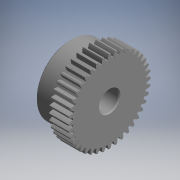
# Autodesk Inventor part: PS1-40_On
Saved by Autodesk Inventor 2017.3 (Build 213256000, 256)
## iProperties
Part Number: PS1-40_On
Material: Generic
Catalog Web Link: www.cadenas.de
Description: Plastic Spur Gears (PS)-
Vendor: KHK
Document SubType Name: Modeling
Designer: partserver
Manufacturer: KHK
Mass: 20.4717 g
Surface Area: 64.8877 cm^2
Volume: 20.4717 cm^3
Density: 1 g/cm^3
Appearance: PSOLRGB-175-175-175
Category: PARTsolutions
Company: KHK
Title: PS1-40
Author: Cadenas PARTsolutions
PSOL_IDENT_0: {$CADENAS_DATA\23d-libs\khk\spur_gears\plastic_spur_gears_ps.prj},178 {VTYP=3D},{NB=PS1-40_On},{LINA=
PSOL_IDENT_1: PS1-40},{NN=Plastic Spur Gears (PS)},{DATE=10.04.2020 06:07:24},{GEOMDATE=05.07.2019 08:26:52},{VERS
PSOL_IDENT_2: ION=},{LINEID=150},{WBVAR=TOOTH},{WBNUMERIC=}  {NB=PS1-40_On},{LINA=PS1-40},{KT=DUMMY},{CN=PS1-40},{
PSOL_IDENT_3: M=1},{MX=1.000},{Z=40},{S=S1},{A=10},{B=35},{C=40.0},{D=42.0},{E=10},{F=10},{G=20},{K=0},{KD=0.0},{M
PSOL_IDENT_4: 1=0},{SCSX=0},{J=0.0},{WMF=S1003.WMF},{R=1.0},{N=0.5},{L=0.1},{L2=0.5},{CBD1=0.0},{CBD2=0.0},{TOOTH=
PSOL_IDENT_5: On}
NB: PS1-40_On
NN: Plastic Spur Gears (PS)
NBSYN: $CN._$TOOTH.
LINA: PS1-40
CATALOG: KHK
CN: PS1-40
M: 1
Z: 40
S: S1
A: 10
B: 35
C: 40
D: 42
E: 10
F: 10
G: 20
K: 0
KD: 0
M1: 0
J: 0
TOOTH: On
SUPPLIER: KHK
ARTICLENO: PS1-40_On
BOMINFO: PS1-40
CREATOR: CADENAS GmbH
Autodesk Inventor part; units mm, degrees
ref_plane "YZ Plane" through (0, 0, 0) normal (1, 0, 0) x (0, 1, 0)
ref_plane "XZ Plane" through (0, 0, 0) normal (0, 1, 0) x (-1, 0, 0)
ref_plane "XY Plane" through (0, 0, 0) normal (0, 0, 1) x (1, 0, 0)
sketch "Sketch_8" plane through (0, 0, 0) normal (0, 0, 1) x (1, 0, 0)
  line L0 (20, 0) -> (0, 0)
  line L1 (0, 5.5) -> (0.5, 5)
  line L2 (0.5, 5) -> (19.5, 5)
  line L3 (19.5, 5) -> (20, 5.5)
  line L4 (20, 5.5) -> (20, 17)
  line L5 (20, 17) -> (19.5, 17.5)
  line L6 (19.5, 17.5) -> (11, 17.5)
  arc A0 (10, 18.5) -> (11, 17.5) centre (11, 18.5) ccw
  line L7 (10, 18.5) -> (10, 20.9)
  line L8 (10, 20.9) -> (9.9, 21)
  line L9 (9.9, 21) -> (0.1, 21)
  line L10 (0.1, 21) -> (0, 20.9)
  line L11 (0, 20.9) -> (0, 5.5)
  constraints: 24 end point, 2 point on circle, 1 centre point
revolve "Revolution1" add sketch "Sketch_8" angle 360 about axis through (20, 0, 0) along (1, 0, 0)
sketch "Sketch_11" plane through (0, 0, 0) normal (1, 0, 0) x (0, 1, 0)
  line L0 (42, 42) -> (-42, 42)
  line L1 (-42, 42) -> (-42, -42)
  line L2 (-42, -42) -> (42, -42)
  line L3 (42, -42) -> (42, 42)
  arc A0 (0.3299, 20.9974) -> (-0.3299, 20.9974) centre (0, 0) ccw
  arc A1 (-0.3299, 20.9974) -> (-1.0303, 18.7217) centre (4.9404, 18.1296) ccw
  arc A2 (-1.0303, 18.7217) -> (-1.9111, 18.6524) centre (0, 0) ccw
  arc A3 (-1.9111, 18.6524) -> (-2.9589, 20.7905) centre (-7.7157, 17.1335) ccw
  arc A4 (-2.9589, 20.7905) -> (-3.6105, 20.6873) centre (0, 0) ccw
  arc A5 (-3.6105, 20.6873) -> (-3.9463, 18.33) centre (2.0435, 18.6792) ccw
  arc A6 (-3.9463, 18.33) -> (-4.8054, 18.1238) centre (0, 0) ccw
  arc A7 (-4.8054, 18.1238) -> (-6.1748, 20.0717) centre (-10.3009, 15.7156) ccw
  arc A8 (-6.1748, 20.0717) -> (-6.8023, 19.8678) centre (0, 0) ccw
  arc A9 (-6.8023, 19.8678) -> (-6.7652, 17.487) centre (-0.9038, 18.7689) ccw
  arc A10 (-6.7652, 17.487) -> (-7.5814, 17.1489) centre (0, 0) ccw
  arc A11 (-7.5814, 17.1489) -> (-9.2387, 18.8586) centre (-12.6326, 13.9107) ccw
  arc A12 (-9.2387, 18.8586) -> (-9.8265, 18.5591) centre (0, 0) ccw
  arc A13 (-9.8265, 18.5591) -> (-9.4175, 16.2134) centre (-3.8287, 18.3965) ccw
  arc A14 (-9.4175, 16.2134) -> (-10.1708, 15.7518) centre (0, 0) ccw
  arc A15 (-10.1708, 15.7518) -> (-12.0751, 17.1811) centre (-14.6532, 11.7632) ccw
  arc A16 (-12.0751, 17.1811) -> (-12.6088, 16.7934) centre (0, 0) ccw
  arc A17 (-12.6088, 16.7934) -> (-11.8379, 14.5405) centre (-6.6594, 17.571) ccw
  arc A18 (-11.8379, 14.5405) -> (-12.5097, 13.9668) centre (0, 0) ccw
  arc A19 (-12.5097, 13.9668) -> (-14.6142, 15.0807) centre (-16.3129, 9.3262) ccw
  arc A20 (-14.6142, 15.0807) -> (-15.0807, 14.6142) centre (0, 0) ccw
  arc A21 (-15.0807, 14.6142) -> (-13.9668, 12.5097) centre (-9.3262, 16.3129) ccw
  arc A22 (-13.9668, 12.5097) -> (-14.5405, 11.8379) centre (0, 0) ccw
  arc A23 (-14.5405, 11.8379) -> (-16.7934, 12.6088) centre (-17.571, 6.6594) ccw
  arc A24 (-16.7934, 12.6088) -> (-17.1811, 12.0751) centre (0, 0) ccw
  arc A25 (-17.1811, 12.0751) -> (-15.7518, 10.1708) centre (-11.7632, 14.6532) ccw
  arc A26 (-15.7518, 10.1708) -> (-16.2134, 9.4175) centre (0, 0) ccw
  arc A27 (-16.2134, 9.4175) -> (-18.5591, 9.8265) centre (-18.3965, 3.8287) ccw
  arc A28 (-18.5591, 9.8265) -> (-18.8586, 9.2387) centre (0, 0) ccw
  arc A29 (-18.8586, 9.2387) -> (-17.1489, 7.5814) centre (-13.9107, 12.6326) ccw
  arc A30 (-17.1489, 7.5814) -> (-17.487, 6.7652) centre (0, 0) ccw
  arc A31 (-17.487, 6.7652) -> (-19.8678, 6.8023) centre (-18.7689, 0.9038) ccw
  arc A32 (-19.8678, 6.8023) -> (-20.0717, 6.1748) centre (0, 0) ccw
  arc A33 (-20.0717, 6.1748) -> (-18.1238, 4.8054) centre (-15.7156, 10.3009) ccw
  arc A34 (-18.1238, 4.8054) -> (-18.33, 3.9463) centre (0, 0) ccw
  arc A35 (-18.33, 3.9463) -> (-20.6873, 3.6105) centre (-18.6792, -2.0435) ccw
  arc A36 (-20.6873, 3.6105) -> (-20.7905, 2.9589) centre (0, 0) ccw
  arc A37 (-20.7905, 2.9589) -> (-18.6524, 1.9111) centre (-17.1335, 7.7157) ccw
  arc A38 (-18.6524, 1.9111) -> (-18.7217, 1.0303) centre (0, 0) ccw
  arc A39 (-18.7217, 1.0303) -> (-20.9974, 0.3299) centre (-18.1296, -4.9404) ccw
  arc A40 (-20.9974, 0.3299) -> (-20.9974, -0.3299) centre (0, 0) ccw
  arc A41 (-20.9974, -0.3299) -> (-18.7217, -1.0303) centre (-18.1296, 4.9404) ccw
  arc A42 (-18.7217, -1.0303) -> (-18.6524, -1.9111) centre (0, 0) ccw
  arc A43 (-18.6524, -1.9111) -> (-20.7905, -2.9589) centre (-17.1335, -7.7157) ccw
  arc A44 (-20.7905, -2.9589) -> (-20.6873, -3.6105) centre (0, 0) ccw
  arc A45 (-20.6873, -3.6105) -> (-18.33, -3.9463) centre (-18.6792, 2.0435) ccw
  arc A46 (-18.33, -3.9463) -> (-18.1238, -4.8054) centre (0, 0) ccw
  arc A47 (-18.1238, -4.8054) -> (-20.0717, -6.1748) centre (-15.7156, -10.3009) ccw
  arc A48 (-20.0717, -6.1748) -> (-19.8678, -6.8023) centre (0, 0) ccw
  arc A49 (-19.8678, -6.8023) -> (-17.487, -6.7652) centre (-18.7689, -0.9038) ccw
  arc A50 (-17.487, -6.7652) -> (-17.1489, -7.5814) centre (0, 0) ccw
  arc A51 (-17.1489, -7.5814) -> (-18.8586, -9.2387) centre (-13.9107, -12.6326) ccw
  arc A52 (-18.8586, -9.2387) -> (-18.5591, -9.8265) centre (0, 0) ccw
  arc A53 (-18.5591, -9.8265) -> (-16.2134, -9.4175) centre (-18.3965, -3.8287) ccw
  arc A54 (-16.2134, -9.4175) -> (-15.7518, -10.1708) centre (0, 0) ccw
  arc A55 (-15.7518, -10.1708) -> (-17.1811, -12.0751) centre (-11.7632, -14.6532) ccw
  arc A56 (-17.1811, -12.0751) -> (-16.7934, -12.6088) centre (0, 0) ccw
  arc A57 (-16.7934, -12.6088) -> (-14.5405, -11.8379) centre (-17.571, -6.6594) ccw
  arc A58 (-14.5405, -11.8379) -> (-13.9668, -12.5097) centre (0, 0) ccw
  arc A59 (-13.9668, -12.5097) -> (-15.0807, -14.6142) centre (-9.3262, -16.3129) ccw
  arc A60 (-15.0807, -14.6142) -> (-14.6142, -15.0807) centre (0, 0) ccw
  arc A61 (-14.6142, -15.0807) -> (-12.5097, -13.9668) centre (-16.3129, -9.3262) ccw
  arc A62 (-12.5097, -13.9668) -> (-11.8379, -14.5405) centre (0, 0) ccw
  arc A63 (-11.8379, -14.5405) -> (-12.6088, -16.7934) centre (-6.6594, -17.571) ccw
  arc A64 (-12.6088, -16.7934) -> (-12.0751, -17.1811) centre (0, 0) ccw
  arc A65 (-12.0751, -17.1811) -> (-10.1708, -15.7518) centre (-14.6532, -11.7632) ccw
  arc A66 (-10.1708, -15.7518) -> (-9.4175, -16.2134) centre (0, 0) ccw
  arc A67 (-9.4175, -16.2134) -> (-9.8265, -18.5591) centre (-3.8287, -18.3965) ccw
  arc A68 (-9.8265, -18.5591) -> (-9.2387, -18.8586) centre (0, 0) ccw
  arc A69 (-9.2387, -18.8586) -> (-7.5814, -17.1489) centre (-12.6326, -13.9107) ccw
  arc A70 (-7.5814, -17.1489) -> (-6.7652, -17.487) centre (0, 0) ccw
  arc A71 (-6.7652, -17.487) -> (-6.8023, -19.8678) centre (-0.9038, -18.7689) ccw
  arc A72 (-6.8023, -19.8678) -> (-6.1748, -20.0717) centre (0, 0) ccw
  arc A73 (-6.1748, -20.0717) -> (-4.8054, -18.1238) centre (-10.3009, -15.7156) ccw
  arc A74 (-4.8054, -18.1238) -> (-3.9463, -18.33) centre (0, 0) ccw
  arc A75 (-3.9463, -18.33) -> (-3.6105, -20.6873) centre (2.0435, -18.6792) ccw
  arc A76 (-3.6105, -20.6873) -> (-2.9589, -20.7905) centre (0, 0) ccw
  arc A77 (-2.9589, -20.7905) -> (-1.9111, -18.6524) centre (-7.7157, -17.1335) ccw
  arc A78 (-1.9111, -18.6524) -> (-1.0303, -18.7217) centre (0, 0) ccw
  arc A79 (-1.0303, -18.7217) -> (-0.3299, -20.9974) centre (4.9404, -18.1296) ccw
  arc A80 (-0.3299, -20.9974) -> (0.3299, -20.9974) centre (0, 0) ccw
  arc A81 (0.3299, -20.9974) -> (1.0303, -18.7217) centre (-4.9404, -18.1296) ccw
  arc A82 (1.0303, -18.7217) -> (1.9111, -18.6524) centre (0, 0) ccw
  arc A83 (1.9111, -18.6524) -> (2.9589, -20.7905) centre (7.7157, -17.1335) ccw
  arc A84 (2.9589, -20.7905) -> (3.6105, -20.6873) centre (0, 0) ccw
  arc A85 (3.6105, -20.6873) -> (3.9463, -18.33) centre (-2.0435, -18.6792) ccw
  arc A86 (3.9463, -18.33) -> (4.8054, -18.1238) centre (0, 0) ccw
  arc A87 (4.8054, -18.1238) -> (6.1748, -20.0717) centre (10.3009, -15.7156) ccw
  arc A88 (6.1748, -20.0717) -> (6.8023, -19.8678) centre (0, 0) ccw
  arc A89 (6.8023, -19.8678) -> (6.7652, -17.487) centre (0.9038, -18.7689) ccw
  arc A90 (6.7652, -17.487) -> (7.5814, -17.1489) centre (0, 0) ccw
  arc A91 (7.5814, -17.1489) -> (9.2387, -18.8586) centre (12.6326, -13.9107) ccw
  arc A92 (9.2387, -18.8586) -> (9.8265, -18.5591) centre (0, 0) ccw
  arc A93 (9.8265, -18.5591) -> (9.4175, -16.2134) centre (3.8287, -18.3965) ccw
  arc A94 (9.4175, -16.2134) -> (10.1708, -15.7518) centre (0, 0) ccw
  arc A95 (10.1708, -15.7518) -> (12.0751, -17.1811) centre (14.6532, -11.7632) ccw
  arc A96 (12.0751, -17.1811) -> (12.6088, -16.7934) centre (0, 0) ccw
  arc A97 (12.6088, -16.7934) -> (11.8379, -14.5405) centre (6.6594, -17.571) ccw
  arc A98 (11.8379, -14.5405) -> (12.5097, -13.9668) centre (0, 0) ccw
  arc A99 (12.5097, -13.9668) -> (14.6142, -15.0807) centre (16.3129, -9.3262) ccw
  arc A100 (14.6142, -15.0807) -> (15.0807, -14.6142) centre (0, 0) ccw
  arc A101 (15.0807, -14.6142) -> (13.9668, -12.5097) centre (9.3262, -16.3129) ccw
  arc A102 (13.9668, -12.5097) -> (14.5405, -11.8379) centre (0, 0) ccw
  arc A103 (14.5405, -11.8379) -> (16.7934, -12.6088) centre (17.571, -6.6594) ccw
  arc A104 (16.7934, -12.6088) -> (17.1811, -12.0751) centre (0, 0) ccw
  arc A105 (17.1811, -12.0751) -> (15.7518, -10.1708) centre (11.7632, -14.6532) ccw
  arc A106 (15.7518, -10.1708) -> (16.2134, -9.4175) centre (0, 0) ccw
  arc A107 (16.2134, -9.4175) -> (18.5591, -9.8265) centre (18.3965, -3.8287) ccw
  arc A108 (18.5591, -9.8265) -> (18.8586, -9.2387) centre (0, 0) ccw
  arc A109 (18.8586, -9.2387) -> (17.1489, -7.5814) centre (13.9107, -12.6326) ccw
  arc A110 (17.1489, -7.5814) -> (17.487, -6.7652) centre (0, 0) ccw
  arc A111 (17.487, -6.7652) -> (19.8678, -6.8023) centre (18.7689, -0.9038) ccw
  arc A112 (19.8678, -6.8023) -> (20.0717, -6.1748) centre (0, 0) ccw
  arc A113 (20.0717, -6.1748) -> (18.1238, -4.8054) centre (15.7156, -10.3009) ccw
  arc A114 (18.1238, -4.8054) -> (18.33, -3.9463) centre (0, 0) ccw
  arc A115 (18.33, -3.9463) -> (20.6873, -3.6105) centre (18.6792, 2.0435) ccw
  arc A116 (20.6873, -3.6105) -> (20.7905, -2.9589) centre (0, 0) ccw
  arc A117 (20.7905, -2.9589) -> (18.6524, -1.9111) centre (17.1335, -7.7157) ccw
  arc A118 (18.6524, -1.9111) -> (18.7217, -1.0303) centre (0, 0) ccw
  arc A119 (18.7217, -1.0303) -> (20.9974, -0.3299) centre (18.1296, 4.9404) ccw
  arc A120 (20.9974, -0.3299) -> (20.9974, 0.3299) centre (0, 0) ccw
  arc A121 (20.9974, 0.3299) -> (18.7217, 1.0303) centre (18.1296, -4.9404) ccw
  arc A122 (18.7217, 1.0303) -> (18.6524, 1.9111) centre (0, 0) ccw
  arc A123 (18.6524, 1.9111) -> (20.7905, 2.9589) centre (17.1335, 7.7157) ccw
  arc A124 (20.7905, 2.9589) -> (20.6873, 3.6105) centre (0, 0) ccw
  arc A125 (20.6873, 3.6105) -> (18.33, 3.9463) centre (18.6792, -2.0435) ccw
  arc A126 (18.33, 3.9463) -> (18.1238, 4.8054) centre (0, 0) ccw
  arc A127 (18.1238, 4.8054) -> (20.0717, 6.1748) centre (15.7156, 10.3009) ccw
  arc A128 (20.0717, 6.1748) -> (19.8678, 6.8023) centre (0, 0) ccw
  arc A129 (19.8678, 6.8023) -> (17.487, 6.7652) centre (18.7689, 0.9038) ccw
  arc A130 (17.487, 6.7652) -> (17.1489, 7.5814) centre (0, 0) ccw
  arc A131 (17.1489, 7.5814) -> (18.8586, 9.2387) centre (13.9107, 12.6326) ccw
  arc A132 (18.8586, 9.2387) -> (18.5591, 9.8265) centre (0, 0) ccw
  arc A133 (18.5591, 9.8265) -> (16.2134, 9.4175) centre (18.3965, 3.8287) ccw
  arc A134 (16.2134, 9.4175) -> (15.7518, 10.1708) centre (0, 0) ccw
  arc A135 (15.7518, 10.1708) -> (17.1811, 12.0751) centre (11.7632, 14.6532) ccw
  arc A136 (17.1811, 12.0751) -> (16.7934, 12.6088) centre (0, 0) ccw
  arc A137 (16.7934, 12.6088) -> (14.5405, 11.8379) centre (17.571, 6.6594) ccw
  arc A138 (14.5405, 11.8379) -> (13.9668, 12.5097) centre (0, 0) ccw
  arc A139 (13.9668, 12.5097) -> (15.0807, 14.6142) centre (9.3262, 16.3129) ccw
  arc A140 (15.0807, 14.6142) -> (14.6142, 15.0807) centre (0, 0) ccw
  arc A141 (14.6142, 15.0807) -> (12.5097, 13.9668) centre (16.3129, 9.3262) ccw
  arc A142 (12.5097, 13.9668) -> (11.8379, 14.5405) centre (0, 0) ccw
  arc A143 (11.8379, 14.5405) -> (12.6088, 16.7934) centre (6.6594, 17.571) ccw
  arc A144 (12.6088, 16.7934) -> (12.0751, 17.1811) centre (0, 0) ccw
  arc A145 (12.0751, 17.1811) -> (10.1708, 15.7518) centre (14.6532, 11.7632) ccw
  arc A146 (10.1708, 15.7518) -> (9.4175, 16.2134) centre (0, 0) ccw
  arc A147 (9.4175, 16.2134) -> (9.8265, 18.5591) centre (3.8287, 18.3965) ccw
  arc A148 (9.8265, 18.5591) -> (9.2387, 18.8586) centre (0, 0) ccw
  arc A149 (9.2387, 18.8586) -> (7.5814, 17.1489) centre (12.6326, 13.9107) ccw
  arc A150 (7.5814, 17.1489) -> (6.7652, 17.487) centre (0, 0) ccw
  arc A151 (6.7652, 17.487) -> (6.8023, 19.8678) centre (0.9038, 18.7689) ccw
  arc A152 (6.8023, 19.8678) -> (6.1748, 20.0717) centre (0, 0) ccw
  arc A153 (6.1748, 20.0717) -> (4.8054, 18.1238) centre (10.3009, 15.7156) ccw
  arc A154 (4.8054, 18.1238) -> (3.9463, 18.33) centre (0, 0) ccw
  arc A155 (3.9463, 18.33) -> (3.6105, 20.6873) centre (-2.0435, 18.6792) ccw
  arc A156 (3.6105, 20.6873) -> (2.9589, 20.7905) centre (0, 0) ccw
  arc A157 (2.9589, 20.7905) -> (1.9111, 18.6524) centre (7.7157, 17.1335) ccw
  arc A158 (1.9111, 18.6524) -> (1.0303, 18.7217) centre (0, 0) ccw
  arc A159 (1.0303, 18.7217) -> (0.3299, 20.9974) centre (-4.9404, 18.1296) ccw
  constraints: 320 point on circle, 160 centre point, 8 end point
extrude "Extrusion1" cut sketch "Sketch_11" along normal blind 10
body "Solid1"
